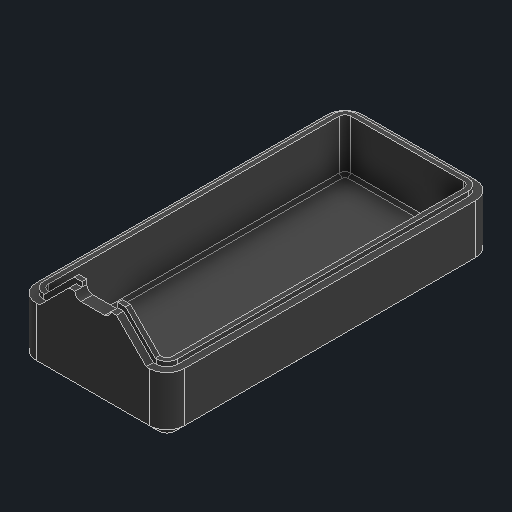
# Autodesk Inventor part: case1
Saved by Autodesk Inventor 2026.2 (Build 302298000, 298)
## iProperties
Created: 2025-12-21
Part Number: case1
Material: Ogólny
Document SubType Name: Modeling
Designer: test
Density: 1 g/cm^3
Appearance: Domyślna
Author: test
## iProperties of the stored document case1_3DPrint.ipt
Created: 2026-01-25
Part Number: case1_3DPrint
Material: Generic
Document SubType Name: Modeling
Designer: mi
Density: 1 g/cm^3
Appearance: Default
Author: mi
Autodesk Inventor part; units mm, degrees
note: some values were not read from the file. Left out: dimensions or parameters whose unit could not be read.
ref_plane "YZ Plane" through (0, 0, 0) normal (1, 0, 0) x (0, 1, 0)
ref_plane "XZ Plane" through (0, 0, 0) normal (0, 1, 0) x (-1, 0, 0)
sketch "Szkic1" plane through (0, 0, 0) normal (0, 1, 0) x (-1, 0, 0)
  line L0 (0, 0) -> (21, 0)
  line L1 (21, 0) -> (21, -51)
  line L2 (21, -51) -> (0, -51)
  line L3 (0, -51) -> (0, 0)
  dimension "d0" = 21
  dimension "d1" = 51
  constraints: 8 end point, 2 parallel, 1 horizontal, 1 perpendicular
  measures "d0" distance between parallel lines of L3 L1
  measures "d1" distance between parallel lines of L2 L0
extrude "Wyciągnięcie proste1" add sketch "Szkic1" along normal blind 8
fillet "Zaokrąglenie1" radius 1 4 edges at (0, 4, 0) (-21, 4, 0) (-21, 4, -51) (0, 4, -51)
chamfer "Chamfer1" distance 0.5 angle 45 8 edges at (0, 0, -25.5) (-0.2929, 0, -50.7071) (-10.5, 0, -51) (-20.7071, 0, -50.7071) (-21, 0, -25.5) (-20.7071, 0, -0.2929) (-10.5, 0, 0) (-0.2929, 0, -0.2929)
shell "Skorupa1" thickness 2 outward yes removed faces 1 at (-7, 8, -17.3333)
sketch "Sketch3" plane through (-20, 8, 2) normal (0, 0, 1) x (1, 0, 0)
  line L0 (19, -8.3284) -> (0, -8.3284) projected
  line L1 (19, 0) -> (19, -8.3284) projected
  line L2 (0, 0) -> (19, 0) projected
  line L3 (0, -8.3284) -> (0, 0) projected
  line L4 (0.5, 0) -> (5.5, 5)
  line L5 (5.5, 5) -> (9.5, 5)
  line L6 (9.5, 0) -> (9.5, 5) construction
  line L7 (18.5, 0) -> (13.5, 5)
  line L8 (13.5, 5) -> (9.5, 5)
  point P0 (20, -8)
  point P1 (18.5, 0)
  dimension "d15" = 5
  dimension "d16" = 8
  dimension "d17" = 5
  constraints: 10 end point, 2 symmetric about line, 1 horizontal, 1 midpoint, 1 point on line, 1 vertical
  measures "d15" horizontal distance of L4.start L4.end
  measures "d16" distance of L4.end L7.end
  measures "d17" distance between parallel lines of L2 L5
extrude "Extrusion3" add sketch "Sketch3" against normal up to surface (2 mm away) contours L2 L4 L5 L8 L7
ref_plane "Work Plane1" through (-10.5, 8, -53) normal (-1, 0, 0) x (0, -1, 0)
sketch "Sketch4" plane through (-10.5, 8, -53) normal (-1, 0, 0) x (0, -1, 0)
  line L0 (0, 0) -> (8.3284, 0) construction
  line L1 (8.3284, 0) -> (0, 0) construction
  line L2 (7.5, 2) -> (0, 2) construction
  line L3 (0, 2) -> (7.5, 2) construction
  line L4 (0, 53) -> (0, 55) projected
  line L5 (0, 52) -> (0, 55) projected
  line L6 (0, 52) -> (0, 3) construction
  line L7 (0, 0) -> (0, 3) construction
  line L8 (0, 3) -> (0, 0) construction
  line L9 (0, 3) -> (0, 52) construction
  line L10 (0, 55) -> (0, 52) projected
  line L11 (0, 55) -> (0, 53) projected
  line L12 (0, 53) -> (0, 52) projected
  line L13 (0, 52) -> (0, 3) construction
  line L14 (0, 3) -> (0, 2) construction
  line L15 (0, 2) -> (0, 3) construction
  line L16 (0, 3) -> (0, 52) construction
  line L17 (0, 52) -> (0, 53) projected
  line L18 (0, 0) -> (-0.8, 0)
  line L19 (-0.8, 0) -> (-0.8, 1.2)
  line L20 (-0.8, 1.2) -> (0, 1.2)
  line L21 (0, 1.2) -> (0, 0)
  line L22 (-0.8, 1.2) -> (0, 1.2)
  line L23 (0, 1.2) -> (0, 2)
  line L24 (0, 2) -> (-0.8, 2)
  line L25 (-0.8, 2) -> (-0.8, 1.2)
  point P0 (8, 53)
  point P1 (0, 1.2)
  dimension "d22" = 0.8
  dimension "d24" = 0.8
  constraints: 16 end point, 4 parallel, 2 horizontal, 2 perpendicular, 1 point on line
  measures "d22" distance between parallel lines of L2 L20
  measures "d24" distance between parallel lines of L21 L19
sketch3d "3D Sketch1"
  line L0 (-1, 8, -51) -> (-20, 8, -51)
  arc A0 (-20, 8, -51) -> (-21, 8, -50) centre (-20, 8, -50) ccw
  line L1 (-21, 8, -50) -> (-21, 8, -1)
  arc A1 (-21, 8, -1) -> (-20, 8, 0) centre (-20, 8, -1) ccw
  line L2 (-20, 8, 0) -> (-19.5, 8, 0)
  line L3 (-19.5, 8, 0) -> (-14.5, 13, 0)
  line L4 (-14.5, 13, 0) -> (-6.5, 13, 0)
  line L5 (-6.5, 13, 0) -> (-1.5, 8, 0)
  line L6 (-1.5, 8, 0) -> (-1, 8, 0)
  arc A2 (-1, 8, 0) -> (0, 8, -1) centre (-1, 8, -1) ccw
  line L7 (0, 8, -1) -> (0, 8, -50)
  arc A3 (0, 8, -50) -> (-1, 8, -51) centre (-1, 8, -50) ccw
sweep "Sweep1" add profiles "Sketch4" path "3D Sketch1" contours L20 L25 L24 L23
sketch "Sketch6" plane through (-20, -0.3284, 2) normal (0, 0, 1) x (1, 0, 0)
  line L0 (19, 0) -> (0, 0) projected
  line L1 (19, 8.3284) -> (19, 0) projected
  line L2 (18.5, 8.3284) -> (19, 8.3284) projected
  line L3 (18.5, 8.3284) -> (13.5, 13.3284) projected
  line L4 (13.5, 13.3284) -> (5.5, 13.3284) projected
  line L5 (5.5, 13.3284) -> (0.5, 8.3284) projected
  line L6 (0, 8.3284) -> (0.5, 8.3284) projected
  line L7 (0, 0) -> (0, 8.3284) projected
  line L8 (7.5, 13.3284) -> (11.5, 13.3284) construction
  line L9 (7.5, 12.3284) -> (11.5, 12.3284)
  line L10 (11.5, 14.3284) -> (7.5, 14.3284)
  arc A0 (7.5, 14.3284) -> (7.5, 12.3284) centre (7.5, 13.3284) ccw
  arc A1 (11.5, 12.3284) -> (11.5, 14.3284) centre (11.5, 13.3284) ccw
  line L11 (5.5, 13.3284) -> (0.5, 8.3284) projected
  line L12 (13.5, 13.3284) -> (5.5, 13.3284) projected
  line L13 (18.5, 8.3284) -> (13.5, 13.3284) projected
  line L14 (19, 8.3284) -> (18.5, 8.3284) projected
  line L15 (19, 9.1284) -> (19, 8.3284) projected
  line L16 (18.8314, 9.1284) -> (19, 9.1284) projected
  line L17 (18.8314, 9.1284) -> (13.8314, 14.1284) projected
  line L18 (13.8314, 14.1284) -> (5.1686, 14.1284) projected
  line L19 (0.1686, 9.1284) -> (5.1686, 14.1284) projected
  line L20 (0, 9.1284) -> (0.1686, 9.1284) projected
  line L21 (0, 9.1284) -> (0, 8.3284) projected
  line L22 (0.5, 8.3284) -> (0, 8.3284) projected
  line L23 (5.1686, 14.1284) -> (13.8314, 14.1284) projected
  line L24 (6.5, 13.3284) -> (12.5, 13.3284)
  line L25 (12.5, 13.3284) -> (12.5, 14.1284)
  line L26 (12.5, 14.1284) -> (6.5, 14.1284)
  line L27 (6.5, 14.1284) -> (6.5, 13.3284)
  point P0 (20, 0.3284)
  point P1 (9.5, 13.3284)
  point P2 (12.5, 14.1284)
  point P3 (12.1, 14.1284)
  point P4 (6.9, 14.1284)
  dimension "d25" = 2
  dimension "d26" = 6
  constraints: 16 end point, 6 point on circle, 4 tangent, 3 parallel, 2 centre point, 2 midpoint, 2 point on line, 1 horizontal, 1 perpendicular
  measures "d25" diameter of A1
  measures "d26" distance of L24.end L24.start
extrude "Extrusion4" cut sketch "Sketch6" against normal up to surface (2 mm away) contours A1 L9 A0 L4 | L4 A0 L18 A1 | A1 L18 L25 | L27 L18 A0 | L18 A0 L10 A1
equation "\"d0\" = case_w"
equation "\"d1\" = case_d"
equation "\"d4\" = wall_thickness"
equation "\"wall_thickness\" = 2"
equation "\"case_w\" = 21"
equation "\"case_d\" = 51"
equation "\"case_h\" = 16"
equation "\"case_mounting\" = 0.8"
